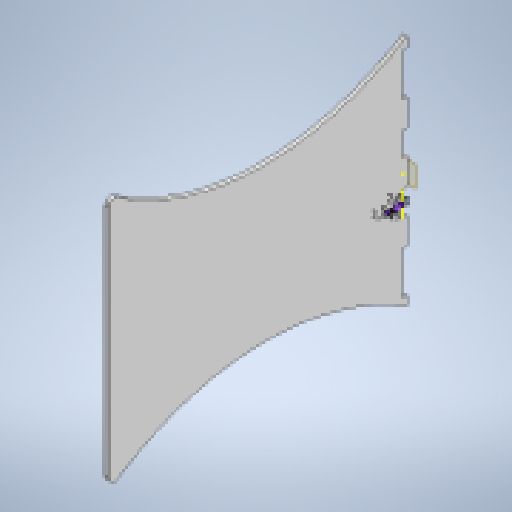
# Autodesk Inventor part: грань тела
Saved by Autodesk Inventor 2023.1 (Build 271208000, 208)
## iProperties
Created: 2024-11-21
Part Number: грань тела
Material: Типовые
Document SubType Name: Modeling
Designer: DELL
Density: 1 g/cm^3
Appearance: По умолчанию
Author: DELL
Autodesk Inventor part; units mm, degrees
ref_plane "YZ Plane" through (0, 0, 0) normal (1, 0, 0) x (0, 1, 0)
ref_plane "XZ Plane" through (0, 0, 0) normal (0, 1, 0) x (-1, 0, 0)
ref_plane "РабПлоскость1" through (0, 0, -4) normal (0, 0, 1) x (1, 0, 0)
sketch "Эскиз10" plane through (0, 0, 0) normal (1, 0, 0) x (0, 1, 0)
  line L0 (-110, -4) -> (110, -4) construction
  line L1 (-120, -4) -> (120, -4) construction
  line L2 (120, -4) -> (120, 276) construction
  line L3 (110.389, 276) -> (-110.389, 276)
  line L4 (-120, 276) -> (-120, -4) construction
  line L5 (-110, -4) -> (110, -4)
  arc A0 (-110, -4) -> (-114.5368, 268.208) centre (-321.9309, 128.6096) ccw
  arc A1 (114.5368, 268.208) -> (110, -4) centre (321.9309, 128.6096) ccw
  arc A2 (114.5368, 268.208) -> (110.389, 276) centre (110.389, 271) ccw
  arc A3 (-110.389, 276) -> (-114.5368, 268.208) centre (-110.389, 271) ccw
  point P0 (0, 0)
  point P1 (0, -4)
  dimension "d50" = 240
  dimension "d51" = 280
  dimension "d52" = 220
  dimension "d53" = 250
  dimension "d54" = 250
  dimension "d55" = 5
  constraints: 10 end point, 10 point on circle, 4 centre point, 4 tangent, 3 midpoint, 2 horizontal, 2 parallel, 2 point on line, 1 equal radius, 1 perpendicular
  measures "d50" distance of L4.start L2.end
  measures "d51" distance of L2.end L1.end
  measures "d52" distance of L5.start L5.end
  measures "d53" radius of A0
  measures "d54" radius of A1
  measures "d55" radius of A2
extrude "Выдавливание6" add sketch "Эскиз10" along normal mid plane 4
sketch "Эскиз12" plane through (2, 0, 0) normal (1, 0, 0) x (0, 0, -1)
  line L0 (4.1067, -100.9593) -> (0, -100.9593)
  line L1 (0, -100.9593) -> (0, -60.9593)
  line L2 (0, -60.9593) -> (4, -60.9593)
  line L3 (4, 110) -> (4, -110) projected
  line L4 (4, -110) -> (4, 110) projected
  line L5 (4, -35.9593) -> (0, -35.9593)
  line L6 (0, -35.9593) -> (0, -12.5)
  line L7 (0, -12.5) -> (4, -12.5)
  line L8 (4, 12.5) -> (0, 12.5)
  line L9 (0, 12.5) -> (0, 35.5004)
  line L10 (0, 35.5004) -> (4, 35.5004)
  line L11 (4, 60.5004) -> (0, 60.5004)
  line L12 (0, 60.5004) -> (0, 100.5004)
  line L13 (0, 100.5004) -> (4, 100.5004)
  point P0 (0, 0)
  point P1 (4, -100.9593)
  constraints: 24 end point, 10 perpendicular, 7 point on line, 2 horizontal, 8 other
extrude "Выдавливание7" cut sketch "Эскиз12" against normal blind 4
sketch "Эскиз13" plane through (2, 0, 0) normal (1, 0, 0) x (0, 0, -1)
  line L0 (-15, -22.6546) -> (-15, -25.8046)
  line L1 (0, -25.7683) -> (0, -22.691)
  line L2 (0, -35.9593) -> (0, -12.5) projected
  line L3 (-6.1608, -27.016) -> (-8.4608, -27.016)
  line L4 (-8.4608, -21.516) -> (-6.1608, -21.516)
  line L5 (-15, -24.2296) -> (0, -24.2296) construction
  line L6 (0, -12.5) -> (0, -35.9593) projected
  line L7 (-8.4608, -27.016) -> (-8.4608, -25.8046)
  line L8 (-8.4608, -22.6546) -> (-8.4608, -21.516)
  line L9 (-15, -25.8046) -> (-8.4608, -25.8046)
  line L10 (-6.1608, -25.7683) -> (0, -25.7683)
  line L11 (-6.1608, -21.516) -> (-6.1608, -22.691)
  line L12 (-6.1608, -25.7683) -> (-6.1608, -27.016)
  line L13 (0, -22.691) -> (-6.1608, -22.691)
  line L14 (-8.4608, -22.6546) -> (-15, -22.6546)
  line L15 (0, 12.5) -> (0, 35.5004) projected
  line L16 (0, 18.7449) -> (0, 30.6124)
  line L17 (0, 22.4252) -> (0, 25.5752)
  line L18 (-15, 25.5752) -> (-15, 22.4252)
  line L19 (-8.65, 21.2502) -> (-6.35, 21.2502)
  line L20 (-6.35, 26.7502) -> (-8.65, 26.7502)
  line L21 (-15, 24.0002) -> (0, 24.0002) construction
  line L22 (-8.65, 26.7502) -> (-8.65, 25.5752)
  line L23 (-8.65, 22.4252) -> (-8.65, 21.2502)
  line L24 (-15, 22.4252) -> (-8.65, 22.4252)
  line L25 (-6.35, 22.4252) -> (0, 22.4252)
  line L26 (-6.35, 21.2502) -> (-6.35, 22.4252)
  line L27 (-6.35, 25.5752) -> (-6.35, 26.7502)
  line L28 (0, 25.5752) -> (-6.35, 25.5752)
  line L29 (-8.65, 25.5752) -> (-15, 25.5752)
  circle A0 centre (-23.1563, -48.4593) radius 9
  line L30 (4, -35.9593) -> (4, -60.9593) projected
  line L31 (4, -48.4593) -> (-57.5802, -48.4593) construction
  line L32 (4, 35.5004) -> (4, 60.5004) projected
  line L33 (0, 0) -> (-64.5188, 0) construction
  circle A1 centre (-23.1563, 48.4593) radius 9
  dimension "d60" = 15
  dimension "d61" = 3.15
  dimension "d62" = 2.3
  dimension "d63" = 5.5
  dimension "d64" = 6.35
  dimension "d70" = 15
  dimension "d71" = 3.15
  dimension "d72" = 2.3
  dimension "d73" = 5.5
  dimension "d77" = 18
  constraints: 58 end point, 20 parallel, 10 perpendicular, 9 midpoint, 8 horizontal, 3 point on line, 2 centre point, 1 symmetric about line, 1 other
  measures "d60" distance of L1.start L0.end
  measures "d61" distance of L0.end L0.start
  measures "d62" distance of L4.start L4.end
  measures "d63" distance of L3.end L4.start
  measures "d64" distance of point (0, -24.23) L11.end
  measures "d70" distance of L18.start L17.end
  measures "d71" distance of L17.end L17.start
  measures "d72" distance of L20.end L20.start
  measures "d73" distance of L20.start L19.end
  measures "d77" diameter of A0
extrude "Выдавливание8" cut sketch "Эскиз13" against normal blind 4
sketch "Эскиз14" plane through (-2, 0, 0) normal (-1, 0, 0) x (0, 0, 1)
  line L0 (71, 37.5) -> (31, 37.5)
  line L1 (26, 32.5) -> (26, -32.5)
  line L2 (31, -37.5) -> (71, -37.5)
  line L3 (76, -32.5) -> (76, 32.5)
  line L4 (0, 0) -> (298.6122, 0) construction
  arc A0 (76, 32.5) -> (71, 37.5) centre (71, 32.5) ccw
  arc A1 (71, -37.5) -> (76, -32.5) centre (71, -32.5) ccw
  arc A2 (31, 37.5) -> (26, 32.5) centre (31, 32.5) ccw
  arc A3 (26, -32.5) -> (31, -37.5) centre (31, -32.5) ccw
  circle A4 centre (71, 32.5) radius 1.575
  circle A5 centre (31, 32.5) radius 1.575
  circle A6 centre (71, -32.5) radius 1.575
  circle A7 centre (31, -32.5) radius 1.575
  circle A8 centre (71, 32.5) radius 5
  circle A9 centre (31, 32.5) radius 5
  circle A10 centre (71, -32.5) radius 5
  circle A11 centre (31, -32.5) radius 5
  line L5 (66, -32.5) -> (36, -32.5)
  line L6 (31, -27.5) -> (31, 27.5)
  line L7 (36, 32.5) -> (66, 32.5)
  line L8 (71, 27.5) -> (71, -27.5)
  line L9 (-4, 12.5) -> (-4, -12.5) projected
  point P0 (26, -37.5)
  point P1 (26, 37.5)
  point P2 (76, -37.5)
  point P3 (76, 0)
  point P4 (31, -37.5)
  point P5 (71, -37.5)
  point P6 (76, -32.5)
  point P7 (76, 32.5)
  point P8 (26, 32.5)
  point P9 (26, -32.5)
  point P10 (71, 37.5)
  point P11 (31, 37.5)
  point P12 (-4, 0)
  dimension "d78" = 50
  dimension "d79" = 75
  dimension "d80" = 5
  dimension "d81" = 3.15
  dimension "d82" = 3.15
  dimension "d83" = 3.15
  dimension "d84" = 3.15
  dimension "d89" = 80
  constraints: 18 end point, 16 point on circle, 12 centre point, 8 coincident, 8 tangent, 7 point on line, 4 parallel, 3 equal radius, 2 horizontal, 2 midpoint, 2 perpendicular
  measures "d78" distance of point (76, -37.5) point (26, -37.5)
  measures "d79" distance of point (26, -37.5) point (26, 37.5)
  measures "d80" radius of A0
  measures "d81" diameter of A4
  measures "d82" diameter of A5
  measures "d83" diameter of A6
  measures "d84" diameter of A7
  measures "d89" distance of point (-4, 0) point (76, 0)
extrude "Выдавливание9" cut sketch "Эскиз14" against normal blind 4 contours L3 A10 L8 A8 | A8 L8 A10 L5 A11 L6 A9 L7 | A9 L6 A11 L1 | A4 | A5 | A6 | A7
